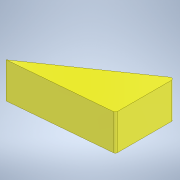
# Autodesk Inventor part: ramp
Saved by Autodesk Inventor 2020 (Build 240168000, 168)
## iProperties
Created: 2020-01-10
Part Number: ramp
Material: Generic
Document SubType Name: Modeling
Designer: xj82b
Density: 1 g/cm^3
Appearance: Yellow
Author: xj82b
Autodesk Inventor part; units mm, degrees
ref_plane "YZ Plane" through (0, 0, 0) normal (1, 0, 0) x (0, 1, 0)
ref_plane "XZ Plane" through (0, 0, 0) normal (0, 1, 0) x (-1, 0, 0)
ref_plane "XY Plane" through (0, 0, 0) normal (0, 0, 1) x (1, 0, 0)
sketch "Sketch1" plane through (0, 0, 0) normal (0, 1, 0) x (-1, 0, 0)
  line L0 (0, 0) -> (90, 0)
  line L1 (90, 0) -> (0, -62)
  line L2 (0, -62) -> (0, 0)
  line L3 (90, 0) -> (0, -8)
  dimension "d8" = 90
  dimension "d9" = 62
  dimension "d10" = 54
  constraints: 8 end point, 1 horizontal, 1 perpendicular, 1 point on line
  measures "d8" distance of L0.start L0.end
  measures "d9" distance of L1.end L0.start
  measures "d10" distance of L3.end L1.end
extrude "Extrusion1" add sketch "Sketch1" along normal blind 32 contours L1 L2 L3
fillet "Fillet3" radius 2 2 edges at (0, 16, -8) (0, 16, -62)
body "Solid1"
